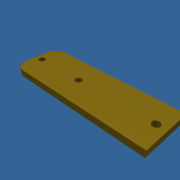
# Autodesk Inventor part: Acrylic_PitchServoSupport_2
Saved by Autodesk Inventor 2012 (Build 160160000, 160)
## iProperties
Created: 2014-03-29
Part Number: Acrylic_PitchServoSupport_2
Material: Default
Document SubType Name: Modeling
Designer: Admin
Density: 1 g/cm^3
Author: Admin
Autodesk Inventor part; units mm, degrees
ref_plane "YZ Plane" through (0, 0, 0) normal (1, 0, 0) x (0, 1, 0)
ref_plane "XZ Plane" through (0, 0, 0) normal (0, 1, 0) x (-1, 0, 0)
ref_plane "XY Plane" through (0, 0, 0) normal (0, 0, 1) x (1, 0, 0)
sketch "Sketch1" plane through (0, 0, 0) normal (0, 0, 1) x (1, 0, 0)
  line L0 (-43.2426, 0) -> (42.2071, 0) projected
  line L1 (0, -15.4497) -> (0, 15.4497) projected
  line L2 (-25, 10) -> (30, 10)
  line L3 (30, 10) -> (30, -10)
  line L4 (30, -10) -> (-25, -10)
  line L5 (-30, -5) -> (-30, 5)
  arc A0 (-25, 10) -> (-30, 5) centre (-25, 5) ccw
  arc A1 (-30, -5) -> (-25, -10) centre (-25, -5) ccw
  point P0 (0, 0)
  point P1 (-30, 10)
  point P2 (-30, -10)
  dimension "d0" = 60
  dimension "d1" = 20
  dimension "d2" = 30
  dimension "d3" = 10
  dimension "d6" = 5
  constraints: 8 end point, 4 point on circle, 4 point on line, 4 tangent, 2 centre point, 2 parallel, 1 equal radius, 1 horizontal, 1 perpendicular
  measures "d0" distance of point (-30, 10) L2.end
  measures "d1" distance of point (-30, -10) point (-30, 10)
  measures "d2" distance between parallel lines of L1 L5
  measures "d3" distance between parallel lines of L0 L2
  measures "d6" radius of A0
extrude "Extrusion1" add sketch "Sketch1" along normal blind 2.8
sketch "Sketch2" plane through (0, 0, 2.8) normal (0, 0, 1) x (1, 0, 0)
  line L0 (30, 10) -> (30, -10) projected
  line L1 (-30, -5) -> (-30, 5) projected
  circle A0 centre (-26.7, 0) radius 1.5
  circle A1 centre (26.2, 0) radius 1.5
  circle A2 centre (-5.65, 0) radius 1.5
  point P0 (0, 0)
  dimension "d7" = 3
  dimension "d8" = 3
  dimension "d9" = 3.8
  dimension "d10" = 3.3
  constraints: 3 centre point, 2 other
  measures "d7" diameter of A0
  measures "d8" diameter of A1
  measures "d9" distance from line of L0 A1.centre
  measures "d10" distance from line of L1 A0.centre
extrude "Extrusion2" cut sketch "Sketch2" against normal blind 10
equation "\"d2\" = 0.5 * d0"
equation "\"d3\" = 0.5 * d1"
body "Solid1"
